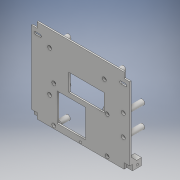
# Autodesk Inventor part: baseplate_odroid_xu4_core
Saved by Autodesk Inventor 2018 (Build 220112000, 112)
## iProperties
Created: 2018-05-14
Part Number: baseplate_odroid_xu4_core
Material: Generic
Document SubType Name: Modeling
Designer: bitbots
Density: 1 g/cm^3
Appearance: Default
Author: bitbots
Autodesk Inventor part; units mm, degrees
ref_plane "YZ Plane" through (0, 0, 0) normal (1, 0, 0) x (0, 1, 0)
ref_plane "XZ Plane" through (0, 0, 0) normal (0, 1, 0) x (-1, 0, 0)
ref_plane "XY Plane" through (0, 0, 0) normal (0, 0, 1) x (1, 0, 0)
sketch "Sketch1" plane through (0, 0, 0) normal (0, 1, 0) x (-1, 0, 0)
  line L0 (-70, 60) -> (70, 60)
  line L1 (70, 60) -> (70, -60)
  line L2 (70, -60) -> (-70, -60)
  line L3 (-70, -60) -> (-70, 60)
  line L4 (-70, 60) -> (70, -60) construction
  line L5 (70, 60) -> (-70, -60) construction
  point P0 (0, 0)
  dimension "d0" = 140
  dimension "d1" = 120
  constraints: 12 end point, 2 midpoint, 2 parallel, 1 horizontal, 1 perpendicular
  measures "d0" distance of L1.end L2.end
  measures "d1" distance of L0.end L1.end
extrude "Extrusion1" add sketch "Sketch1" along normal blind 2
sketch "Sketch6" plane through (0, 2, 0) normal (0, 1, 0) x (1, 0, 0)
  line L0 (-70, -60) -> (70, -60) projected
  line L1 (70, -60) -> (70, 60) projected
  line L2 (70, 60) -> (-70, 60) projected
  line L3 (-70, 60) -> (-70, -60) projected
  line L4 (70, 60) -> (70, -60) projected
  line L5 (70, 60) -> (60, 60)
  line L6 (60, 60) -> (60, 50)
  line L7 (60, 50) -> (70, 50)
  line L8 (70, 50) -> (70, 60)
  point P0 (0, 0)
  dimension "d49" = 10
  dimension "d50" = 10
  constraints: 8 end point, 2 parallel, 1 horizontal, 1 perpendicular
  measures "d49" distance of L7.end L6.end
  measures "d50" distance of L6.end L5.end
extrude "Extrusion6" add sketch "Sketch6" along normal blind 15 contours L7 L6 L2 L1
sketch "Sketch8" plane through (70, 0, 60) normal (1, 0, 0) x (0, 0, -1)
  line L0 (120, 0) -> (0, 0) projected
  line L1 (120, 0) -> (120, 17) projected
  line L2 (110, 17) -> (120, 17) projected
  line L3 (110, 2) -> (110, 17) projected
  line L4 (0, 2) -> (110, 2) projected
  line L5 (0, 0) -> (0, 2) projected
  line L6 (110, 2) -> (110, 11)
  line L7 (110, 2) -> (110, 17) projected
  line L8 (110, 11) -> (116, 11)
  circle A0 centre (116, 11) radius 1.5
  point P0 (60, 0)
  dimension "d56" = 9
  dimension "d57" = 6
  dimension "d58" = 3
  constraints: 4 end point, 1 centre point, 1 coincident, 1 perpendicular, 1 point on line
  measures "d56" distance of L3.start L6.end
  measures "d57" distance of L6.end L8.end
  measures "d58" diameter of A0
extrude "Extrusion8" cut sketch "Sketch8" against normal blind 10 contours A0
mirror "Mirror1" about plane through (0, 0, 0) normal (1, 0, 0) of "Extrusion6", "Extrusion8"
chamfer "Chamfer1" distance 8 angle 45 4 edges at (-60, 2, -55) (60, 2, -55) (-65, 2, -50) (65, 2, -50)
sketch "Sketch9" plane through (0, 0, 0) normal (0, -1, 0) x (1, 0, 0)
  line L0 (70, 60) -> (-70, 60) projected
  line L1 (-70, 60) -> (-70, -60) projected
  line L2 (-70, -60) -> (70, -60) projected
  line L3 (70, -60) -> (70, 60) projected
  line L4 (-70, 60) -> (-70, -60) projected
  line L5 (-70, -60) -> (-62, -60)
  line L6 (-62, -60) -> (-62, -52)
  line L7 (-62, -52) -> (-70, -52)
  line L8 (-70, -52) -> (-70, -60)
  line L9 (70, -60) -> (60, -60) projected
  line L10 (70, -60) -> (60, -60)
  line L11 (70, -50) -> (70, -60)
  line L12 (70, 60) -> (62, 60)
  line L13 (62, 60) -> (62, 52)
  line L14 (62, 52) -> (70, 52)
  line L15 (70, 52) -> (70, 60)
  line L16 (70, 60) -> (-70, 60) projected
  line L17 (-70, 60) -> (-62, 60)
  line L18 (-62, 60) -> (-62, 52)
  line L19 (-62, 52) -> (-70, 52)
  line L20 (-70, 52) -> (-70, 60)
  line L21 (70, -60) -> (62, -60)
  line L22 (62, -60) -> (62, -52)
  line L23 (62, -52) -> (70, -52)
  line L24 (70, -52) -> (70, -60)
  point P0 (0, 0)
  dimension "d64" = 8
  dimension "d65" = 8
  dimension "d68" = 8
  dimension "d69" = 8
  dimension "d70" = 8
  dimension "d71" = 8
  dimension "d96" = 8
  dimension "d97" = 8
  constraints: 36 end point, 8 parallel, 5 horizontal, 4 perpendicular
  measures "d64" distance of L7.end L6.end
  measures "d65" distance of L6.end L5.end
  measures "d68" distance of L14.end L13.end
  measures "d69" distance of L13.end L12.end
  measures "d70" distance of L18.end L19.end
  measures "d71" distance of L17.end L18.end
  measures "d96" distance of L22.end L23.end
  measures "d97" distance of L21.end L22.end
extrude "Extrusion9" cut sketch "Sketch9" against normal blind 4 contours L3 L14 L13 L0 | L18 L19 L1 L0 | L3 L2 L22 L23 | L7 L6 L2 L1
sketch "Sketch10" plane through (0, 2, 0) normal (0, 1, 0) x (1, 0, 0)
  line L0 (-62, -60) -> (62, -60) projected
  line L1 (70, -52) -> (70, 42) projected
  line L2 (52, 42) -> (70, 42) projected
  line L3 (52, 60) -> (52, 42) projected
  line L4 (52, 60) -> (-52, 60) projected
  line L5 (-52, 42) -> (-52, 60) projected
  line L6 (-70, 42) -> (-52, 42) projected
  line L7 (-70, 42) -> (-70, -52) projected
  line L8 (-70, 60) -> (70, 60) projected
  line L9 (0, 60) -> (0, 57.5)
  circle A0 centre (0, 57.5) radius 1.5
  line L10 (62, -52) -> (70, -52) projected
  line L11 (-70, -52) -> (-62, -52) projected
  line L12 (-62, -52) -> (-62, -60) projected
  line L13 (62, -60) -> (62, -52) projected
  point P0 (0, 0)
  point P1 (-62, 60)
  point P2 (60, 60)
  dimension "d74" = 2.5
  dimension "d75" = 3
  constraints: 2 end point, 1 centre point, 1 coincident, 1 midpoint, 1 vertical
  measures "d74" distance of L9.start L9.end
  measures "d75" diameter of A0
extrude "Extrusion10" cut sketch "Sketch10" against normal blind 4 contours A0
sketch "Sketch13" plane through (0, 2, 0) normal (0, 1, 0) x (1, 0, 0)
  line L0 (-62, -60) -> (62, -60) projected
  line L1 (70, -52) -> (70, 42) projected
  line L2 (52, 42) -> (70, 42) projected
  line L3 (52, 60) -> (52, 42) projected
  line L4 (52, 60) -> (-52, 60) projected
  line L5 (-52, 42) -> (-52, 60) projected
  line L6 (-70, 42) -> (-52, 42) projected
  line L7 (-70, 42) -> (-70, -52) projected
  circle A0 centre (0, 57.5) radius 1.5 projected
  line L8 (-70, -60) -> (-61, -60)
  line L9 (-62, -60) -> (62, -60) projected
  line L10 (-61, -60) -> (-61, -45)
  line L11 (-64.5, -45) -> (-57.5, -45) construction
  line L12 (-64.5, -46.75) -> (-57.5, -46.75)
  line L13 (-57.5, -43.25) -> (-64.5, -43.25)
  arc A1 (-64.5, -43.25) -> (-64.5, -46.75) centre (-64.5, -45) ccw
  arc A2 (-57.5, -46.75) -> (-57.5, -43.25) centre (-57.5, -45) ccw
  line L14 (-70, -52) -> (-62, -52) projected
  line L15 (-62, -52) -> (-62, -60) projected
  line L16 (62, -60) -> (62, -52) projected
  line L17 (62, -52) -> (70, -52) projected
  point P0 (0, 0)
  dimension "d90" = 9
  dimension "d91" = 15
  dimension "d92" = 3.5
  dimension "d93" = 3.5
  constraints: 12 end point, 4 point on circle, 4 tangent, 2 centre point, 1 collinear, 1 horizontal, 1 midpoint, 1 parallel, 1 perpendicular
  measures "d90" distance of L8.start L8.end
  measures "d91" distance of L8.end L10.end
  measures "d92" distance of L10.end L11.end
  measures "d93" diameter of A2
extrude "Extrusion13" cut sketch "Sketch13" against normal blind 3 contours A1 L13 A2 L12
mirror "Mirror3" about plane through (0, 0, 0) normal (1, 0, 0) of "Extrusion13"
sketch "Sketch25" plane through (0, 2, 0) normal (0, 1, 0) x (1, 0, 0)
  line L0 (52, 60) -> (-52, 60) construction
  line L1 (-52, 42) -> (-52, 60) construction
  line L2 (-70, 42) -> (-52, 42) construction
  line L3 (-70, 42) -> (-70, -52) construction
  line L4 (-70, -52) -> (-62, -52) construction
  line L5 (-62, -52) -> (-62, -60) construction
  line L6 (-62, -60) -> (62, -60) construction
  line L7 (62, -60) -> (62, -52) construction
  line L8 (62, -52) -> (70, -52) construction
  line L9 (70, -52) -> (70, 42) construction
  line L10 (52, 42) -> (70, 42) construction
  line L11 (52, 60) -> (52, 42) construction
  arc A0 (57.5, -43.25) -> (57.5, -46.75) centre (57.5, -45) ccw construction
  line L12 (57.5, -43.25) -> (64.5, -43.25) construction
  arc A1 (64.5, -46.75) -> (64.5, -43.25) centre (64.5, -45) ccw construction
  line L13 (64.5, -46.75) -> (57.5, -46.75) construction
  arc A2 (-57.5, -46.75) -> (-57.5, -43.25) centre (-57.5, -45) ccw construction
  line L14 (-57.5, -46.75) -> (-64.5, -46.75) construction
  arc A3 (-64.5, -43.25) -> (-64.5, -46.75) centre (-64.5, -45) ccw construction
  line L15 (-64.5, -43.25) -> (-57.5, -43.25) construction
  circle A4 centre (0, 57.5) radius 1.5 construction
  line L16 (61, -9) -> (61, 21) construction
  circle A5 centre (61, 21) radius 1.6
  circle A6 centre (61, -9) radius 1.6
  line L17 (0, 0) -> (0, -80) construction
  line L18 (0, 0) -> (80, 0) construction
  circle A7 centre (-44, 21) radius 1.6
  circle A8 centre (-44, -37) radius 1.6
  circle A9 centre (34, -37) radius 1.6
  line L19 (62, -52) -> (62, -37)
  line L20 (64.5, -46.75) -> (57.5, -46.75) projected
  line L21 (62, -52) -> (77, -52) construction
  line L22 (62, -37) -> (-44, -37)
  line L23 (-44, -37) -> (-44, 21)
  line L24 (-44, 21) -> (61, 21)
  line L25 (-44, -37) -> (34, -37)
  line L26 (62, -52) -> (70, -52) projected
  line L27 (70, -52) -> (70, -37)
  line L28 (70, 52) -> (70, -52) projected
  line L29 (70, -52) -> (85, -52) construction
  line L30 (70, -37) -> (62, -37)
  dimension "d148" = 30
  dimension "d150" = 3.2
  dimension "d151" = 3.2
  dimension "d152" = 80
  dimension "d153" = 90
  dimension "d155" = 3.2
  dimension "d246" = 15
  dimension "d247" = 90
  dimension "d248" = 106
  dimension "d249" = 58
  dimension "d250" = 105
  dimension "d251" = 78
  dimension "d263" = 8
  dimension "d266" = 15
  dimension "d267" = 90
  constraints: 24 end point, 5 centre point, 5 coincident, 5 horizontal, 4 perpendicular, 3 vertical, 2 collinear, 1 point on line
  measures "d148" distance of L16.end L16.start
  measures "d150" diameter of A5
  measures "d151" diameter of A6
  measures "d152" distance of L17.start L17.end
  measures "d153" angle of L17 L18
  measures "d155" diameter of A9
  measures "d246" distance of L19.start L19.end
  measures "d247" angle of L21 L19
  measures "d248" distance of L19.end L22.end
  measures "d249" distance of L22.end L23.end
  measures "d250" distance of L23.end L16.end
  measures "d251" distance of L22.end L25.end
  measures "d263" distance from line of L9 L19.end
  measures "d266" distance of L8.end L27.end
  measures "d267" angle of L29 L27
extrude "Extrusion22" cut sketch "Sketch25" against normal blind 10 contours A5 | A6 | L24 L23 A7 | A7 L23 L24 | L22 L23 A8 | A8 L23 L22 | L22 A9 | A9 L22
sketch "Sketch26" plane through (0, 2, 0) normal (0, 1, 0) x (1, 0, 0)
  circle A0 centre (-44, 21) radius 1.6 projected
  circle A1 centre (61, -9) radius 1.6 construction
  circle A2 centre (61, 21) radius 1.6 construction
  circle A3 centre (-44, -37) radius 1.6 projected
  circle A4 centre (34, -37) radius 1.6 construction
  circle A5 centre (0, 57.5) radius 1.5 construction
  arc A6 (-57.5, -46.75) -> (-57.5, -43.25) centre (-57.5, -45) ccw construction
  line L0 (-57.5, -46.75) -> (-64.5, -46.75) construction
  arc A7 (-64.5, -43.25) -> (-64.5, -46.75) centre (-64.5, -45) ccw construction
  line L1 (-64.5, -43.25) -> (-57.5, -43.25) construction
  arc A8 (57.5, -43.25) -> (57.5, -46.75) centre (57.5, -45) ccw construction
  line L2 (57.5, -43.25) -> (64.5, -43.25) construction
  arc A9 (64.5, -46.75) -> (64.5, -43.25) centre (64.5, -45) ccw construction
  line L3 (64.5, -46.75) -> (57.5, -46.75) construction
  line L4 (52, 60) -> (-52, 60) construction
  line L5 (-52, 42) -> (-52, 60) construction
  line L6 (-70, 42) -> (-52, 42) construction
  line L7 (-70, 42) -> (-70, -52) construction
  line L8 (-70, -52) -> (-62, -52) construction
  line L9 (-62, -52) -> (-62, -60) construction
  line L10 (-62, -60) -> (62, -60) construction
  line L11 (62, -60) -> (62, -52) construction
  line L12 (62, -52) -> (70, -52) construction
  line L13 (70, -52) -> (70, 42) construction
  line L14 (52, 42) -> (70, 42) construction
  line L15 (52, 60) -> (52, 42) construction
  circle A10 centre (-44, -37) radius 1.6 construction
  circle A11 centre (-44, -37) radius 3.5
  circle A12 centre (-44, 21) radius 3.5
  circle A13 centre (61, -9) radius 1.6 projected
  circle A14 centre (61, -9) radius 3.5
  circle A15 centre (61, 21) radius 1.6 projected
  circle A16 centre (61, 21) radius 3.5
  circle A17 centre (34, -37) radius 1.6 projected
  circle A18 centre (34, -37) radius 3.5
  point P0 (0, 0)
  dimension "d158" = 7
  dimension "d159" = 7
  dimension "d160" = 7
  dimension "d161" = 7
  dimension "d162" = 7
  constraints: 5 centre point, 5 coincident
  measures "d158" diameter of A11
  measures "d159" diameter of A12
  measures "d160" diameter of A14
  measures "d161" diameter of A16
  measures "d162" diameter of A18
extrude "Extrusion23" add sketch "Sketch26" along normal blind 25
sketch "Sketch27" plane through (0, 0, 0) normal (0, -1, 0) x (1, 0, 0)
  circle A0 centre (-44, -21) radius 1.6 construction
  circle A1 centre (61, 9) radius 1.6 construction
  circle A2 centre (61, -21) radius 1.6 construction
  circle A3 centre (-44, 37) radius 1.6 construction
  circle A4 centre (34, 37) radius 1.6 construction
  arc A5 (57.5, 46.75) -> (57.5, 43.25) centre (57.5, 45) ccw construction
  line L0 (57.5, 46.75) -> (64.5, 46.75) construction
  arc A6 (64.5, 43.25) -> (64.5, 46.75) centre (64.5, 45) ccw construction
  line L1 (64.5, 43.25) -> (57.5, 43.25) construction
  arc A7 (-57.5, 43.25) -> (-57.5, 46.75) centre (-57.5, 45) ccw construction
  line L2 (-57.5, 43.25) -> (-64.5, 43.25) construction
  arc A8 (-64.5, 46.75) -> (-64.5, 43.25) centre (-64.5, 45) ccw construction
  line L3 (-64.5, 46.75) -> (-57.5, 46.75) construction
  circle A9 centre (0, -57.5) radius 1.5 construction
  line L4 (-62, -52) -> (-62, -60) construction
  line L5 (-62, -60) -> (62, -60) construction
  line L6 (62, -60) -> (62, -52) construction
  line L7 (62, -52) -> (70, -52) construction
  line L8 (70, -52) -> (70, 52) construction
  line L9 (70, 52) -> (62, 52) construction
  line L10 (62, 52) -> (62, 60) construction
  line L11 (62, 60) -> (-62, 60) construction
  line L12 (-62, 60) -> (-62, 52) construction
  line L13 (-62, 52) -> (-70, 52) construction
  line L14 (-70, 52) -> (-70, -52) construction
  line L15 (-70, -52) -> (-62, -52) construction
  circle A10 centre (61, 9) radius 1.6 construction
  circle A11 centre (61, 9) radius 2.8
  circle A12 centre (61, -21) radius 2.8
  circle A13 centre (34, 37) radius 1.6 projected
  circle A14 centre (34, 37) radius 2.8
  circle A15 centre (-44, 37) radius 1.6 projected
  circle A16 centre (-44, 37) radius 2.8
  circle A17 centre (-44, -21) radius 1.6 projected
  circle A18 centre (-44, -21) radius 2.8
  point P0 (0, 0)
  dimension "d165" = 5.6
  dimension "d166" = 5.6
  dimension "d167" = 5.6
  dimension "d168" = 5.6
  dimension "d169" = 5.6
  constraints: 5 centre point, 5 coincident
  measures "d165" diameter of A11
  measures "d166" diameter of A12
  measures "d167" diameter of A14
  measures "d168" diameter of A16
  measures "d169" diameter of A18
extrude "Extrusion24" cut sketch "Sketch27" against normal blind 3
sketch "Sketch30" plane through (0, 2, 0) normal (0, 1, 0) x (1, 0, 0)
  line L0 (38, 56) -> (38, 4) construction
  line L1 (38, 4) -> (-38, 4) construction
  line L2 (-38, 4) -> (-38, 56) construction
  line L3 (-38, 56) -> (38, 56) construction
  circle A0 centre (38, 4) radius 1.75
  circle A1 centre (38, 56) radius 1.75
  circle A2 centre (38, 4) radius 3.5
  circle A3 centre (38, 56) radius 3.5
  line L4 (0, 4) -> (0, 56) construction
  circle A4 centre (0, 57.5) radius 1.5 construction
  circle A5 centre (-38, 4) radius 1.75
  circle A6 centre (-38, 56) radius 1.75
  circle A7 centre (-38, 4) radius 3.5
  circle A8 centre (-38, 56) radius 3.5
  point P0 (0, 0)
  dimension "d226" = 52
  dimension "d227" = 76
  dimension "d228" = 52
  dimension "d229" = 3.5
  dimension "d230" = 3.5
  dimension "d231" = 7
  dimension "d232" = 7
  constraints: 10 end point, 8 centre point, 6 coincident, 4 symmetric about line, 2 midpoint, 2 perpendicular, 1 horizontal, 1 vertical alignment, 5 other
  measures "d226" distance of L0.start L0.end
  measures "d227" distance of L0.end L1.end
  measures "d228" distance of L1.end L2.end
  measures "d229" diameter of A0
  measures "d230" diameter of A1
  measures "d231" diameter of A2
  measures "d232" diameter of A3
extrude "Extrusion27" add sketch "Sketch30" along normal blind 18
sketch "Sketch31" plane through (0, 0, 0) normal (0, -1, 0) x (1, 0, 0)
  circle A0 centre (38, -56) radius 2.8
  circle A1 centre (38, -4) radius 2.8
  circle A2 centre (-38, -56) radius 2.8
  circle A3 centre (-38, -4) radius 2.8
  point P0 (0, 0)
  dimension "d235" = 5.6
  dimension "d236" = 5.6
  dimension "d237" = 5.6
  dimension "d238" = 5.6
  constraints: 8 coincident, 4 centre point
  measures "d235" diameter of A0
  measures "d236" diameter of A1
  measures "d237" diameter of A2
  measures "d238" diameter of A3
extrude "Extrusion28" cut sketch "Sketch31" against normal blind 3
chamfer "Chamfer5" distance 5 angle 45 4 edges at (-41.5, 2, -56) (34.5, 2, -56) (34.5, 2, -4) (-41.5, 2, -4)
chamfer "Chamfer6" distance 5 angle 45 5 edges at (-47.5, 2, 37) (-47.5, 2, -21) (30.5, 2, 37) (57.5, 2, 9) (57.5, 2, -21)
sketch "Sketch32" plane through (0, 2, 0) normal (0, 1, 0) x (1, 0, 0)
  circle A0 centre (61, -9) radius 8.5 construction
  circle A1 centre (-44, 21) radius 8.5 construction
  circle A2 centre (-44, -37) radius 8.5 construction
  arc A3 (-57.5, -46.75) -> (-57.5, -43.25) centre (-57.5, -45) ccw construction
  line L0 (-57.5, -46.75) -> (-64.5, -46.75) construction
  arc A4 (-64.5, -43.25) -> (-64.5, -46.75) centre (-64.5, -45) ccw construction
  line L1 (-64.5, -43.25) -> (-57.5, -43.25) construction
  circle A5 centre (38, 4) radius 8.5 construction
  arc A6 (30.5, 60) -> (45.5, 60) centre (38, 56) ccw construction
  line L2 (30.5, 60) -> (-30.5, 60) construction
  arc A7 (-45.5, 60) -> (-30.5, 60) centre (-38, 56) ccw construction
  line L3 (-45.5, 60) -> (-52, 60) construction
  line L4 (-52, 42) -> (-52, 60) construction
  line L5 (-70, 42) -> (-52, 42) construction
  line L6 (-70, 42) -> (-70, -52) construction
  line L7 (-70, -52) -> (-62, -52) construction
  line L8 (-62, -52) -> (-62, -60) construction
  line L9 (-62, -60) -> (62, -60) construction
  line L10 (62, -60) -> (62, -52) construction
  line L11 (62, -52) -> (70, -52) construction
  line L12 (52, 42) -> (70, 42) construction
  line L13 (52, 60) -> (52, 42) construction
  line L14 (52, 60) -> (45.5, 60) construction
  arc A8 (57.5, -43.25) -> (57.5, -46.75) centre (57.5, -45) ccw construction
  line L15 (57.5, -43.25) -> (64.5, -43.25) construction
  arc A9 (64.5, -46.75) -> (64.5, -43.25) centre (64.5, -45) ccw construction
  line L16 (64.5, -46.75) -> (57.5, -46.75) construction
  circle A10 centre (0, 57.5) radius 1.5 construction
  circle A11 centre (-38, 4) radius 8.5 construction
  circle A12 centre (34, -37) radius 8.5 construction
  circle A13 centre (61, 21) radius 8.5 construction
  circle A14 centre (-38, 56) radius 1.75 construction
  line L17 (-38, 56) -> (-38, 51) construction
  line L18 (-38, 51) -> (-33, 51) construction
  line L19 (-33, 51) -> (7, 51)
  line L20 (7, 51) -> (7, 11)
  line L21 (7, 11) -> (-33, 11)
  line L22 (-33, 11) -> (-33, 51)
  circle A15 centre (-44, 21) radius 1.6 construction
  line L23 (-44, 21) -> (61, 21) construction
  line L24 (8.5, 21) -> (8.5, -37) construction
  line L25 (-16.5, 4.5) -> (33.5, 4.5)
  line L26 (33.5, 4.5) -> (33.5, -20.5)
  line L27 (33.5, -20.5) -> (-16.5, -20.5)
  line L28 (-16.5, -20.5) -> (-16.5, 4.5)
  line L29 (-16.5, 4.5) -> (33.5, -20.5) construction
  line L30 (33.5, 4.5) -> (-16.5, -20.5) construction
  line L31 (70, -52) -> (70, 42) projected
  point P0 (0, 0)
  point P1 (8.5, -8)
  dimension "d255" = 5
  dimension "d256" = 5
  dimension "d257" = 40
  dimension "d258" = 40
  dimension "d259" = 50
  dimension "d260" = 25
  constraints: 28 end point, 4 midpoint, 4 parallel, 3 horizontal, 3 perpendicular, 2 vertical
  measures "d255" distance of L17.start L17.end
  measures "d256" distance of L17.end L18.end
  measures "d257" distance of L20.end L21.end
  measures "d258" distance of L19.end L20.end
  measures "d259" distance of L26.end L27.end
  measures "d260" distance of L25.end L26.end
extrude "Extrusion29" cut sketch "Sketch32" against normal blind 3
body "Solid1"
